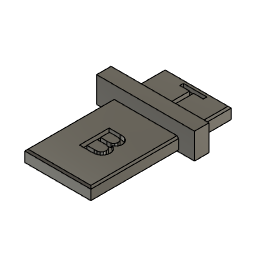
Micro-SD Slot Cover v4 (Autodesk Fusion 360 design; units mm, degrees)
Autodesk Fusion 360 part; units mm, degrees
sketch "Sketch1" plane through (0, 0, 0) normal (0, 1, 0) x (1, 0, 0)
  line L0 (-40, -20) -> (-32, -20)
  line L1 (-32, -20) -> (-32, -18.4)
  line L2 (-32, -18.4) -> (-40, -18.4)
  line L3 (-40, -18.4) -> (-40, -20)
  dimension "d1" = 8
  dimension "d2" = 1.6
  constraint horizontal L0
  constraint vertical L1
  constraint horizontal L2
  constraint vertical L3
  measures "d1" distance of L0.start L0.end
  measures "d2" distance of L0.end L1.end
extrude "Extrude1" add sketch "Sketch1" along normal blind 17 makes body 1
sketch "Sketch2" plane through (0, 0, 20) normal (0, 0, 1) x (-1, 0, 0)
  line L0 (40, 0) -> (32, 0)
  line L1 (32, 0) -> (32, -17)
  line L2 (32, -17) -> (40, -17)
  line L3 (40, -17) -> (40, 0)
  line L4 (42.4149, -10.625) -> (29.5, -10.625) construction
  line L5 (42.5, -12.575) -> (29.2903, -12.575) construction
  line L6 (41.928, -12.575) -> (30.072, -12.575)
  line L7 (30.072, -12.575) -> (30.072, -10.625)
  line L8 (30.072, -10.625) -> (41.928, -10.625)
  line L9 (41.928, -10.625) -> (41.928, -12.575)
  dimension "d5" = 10.625
  dimension "d6" = 12.575
  dimension "d7" = 11.856
  dimension "d8" = 1.928
  constraint perpendicular L3 L4
  constraint perpendicular L3 L5
  constraint horizontal L6
  constraint vertical L7
  constraint horizontal L8
  constraint vertical L9
  constraint coincident L4 L7.end
  measures "d5" distance of L0.start L4
  measures "d6" distance of L0.start L5
  measures "d7" distance of L6.start L6.end
  measures "d8" distance of L3 L9
extrude "Extrude2" add sketch "Sketch2" along normal blind 1.534 separate body contours L3 L6 L8 L9 | L1 L3 L6 L8 | L1 L6 L7 L8 makes body 2
extrude "Extrude3" add sketch "Sketch2" against normal blind 1.6 contours L1 L6 L7 L8 bodies 1 2
extrude "Extrude4" add sketch "Sketch2" against normal blind 1.6 contours L3 L6 L8 L9 bodies 1
sketch "Sketch3" plane through (0, 0, 20) normal (0, 0, 1) x (1, 0, 0)
  line L0 (-37.1233, 3.7297) -> (-34.4207, 3.7297) construction
  line L1 (-34.4207, 3.7297) -> (-34.4207, 8.7297) construction
  line L2 (-34.4207, 8.7297) -> (-37.1233, 8.7297) construction
  line L3 (-37.1233, 8.7297) -> (-37.1233, 3.7297) construction
  line L4 (-37.2983, 12.9016) -> (-34.4613, 12.9016) construction
  line L5 (-34.4613, 12.9016) -> (-34.4613, 17.9016) construction
  line L6 (-34.4613, 17.9016) -> (-37.2983, 17.9016) construction
  line L7 (-37.2983, 17.9016) -> (-37.2983, 12.9016) construction
  text T0 "B" font "Arial" height 5 align ink ink in box 0 x 0 at (-37.1233, 3.7297) x (1, 0) y (0, 1) spacing 1 height is em
  text T1 "T" font "Arial" height 5 align ink ink in box 0 x 0 at (-37.2983, 12.9016) x (1, 0) y (0, 1) spacing 1 height is em
  constraint perpendicular L0 L1
  constraint parallel L0 L2
  constraint parallel L1 L3
  constraint perpendicular L4 L5
  constraint parallel L4 L6
  constraint parallel L5 L7
extrude "Extrude5" cut sketch "Sketch3" against normal blind 0.5 text T0 bodies 1
extrude "Extrude6" cut sketch "Sketch3" against normal blind 0.5 text T1 bodies 1
chamfer "Chamfer1" distance 0.2 angle 45 1 edges at (-32, 14.7875, 18.4) on bodies 1
chamfer "Chamfer2" distance 0.2 angle 45 1 edges at (-32, 5.3125, 18.4) on bodies 1
chamfer "Chamfer3" distance 0.2 angle 45 1 edges at (-32, 14.7875, 20) on bodies 1
chamfer "Chamfer4" distance 0.2 angle 45 1 edges at (-32, 5.3125, 20) on bodies 1
chamfer "Chamfer5" distance 0.2 angle 45 1 edges at (-40, 14.7875, 18.4) on bodies 1
chamfer "Chamfer6" distance 0.2 angle 45 1 edges at (-40, 14.7875, 20) on bodies 1
chamfer "Chamfer7" distance 0.2 angle 45 1 edges at (-40, 5.3125, 20) on bodies 1
chamfer "Chamfer8" distance 0.2 angle 45 1 edges at (-40, 5.3125, 18.4) on bodies 1
chamfer "Chamfer9" distance 0.2 angle 45 1 edges at (-36, 17, 20) on bodies 1
chamfer "Chamfer10" distance 0.2 angle 45 1 edges at (-36, 17, 18.4) on bodies 1
chamfer "Chamfer11" distance 0.2 angle 45 1 edges at (-36, 0, 20) on bodies 1
chamfer "Chamfer12" distance 0.2 angle 45 1 edges at (-36, 0, 18.4) on bodies 1
move_face "OffsetFaces1" offset -0.2 1 faces at (-37.2667, 12.575, 21.0227) on bodies 1
